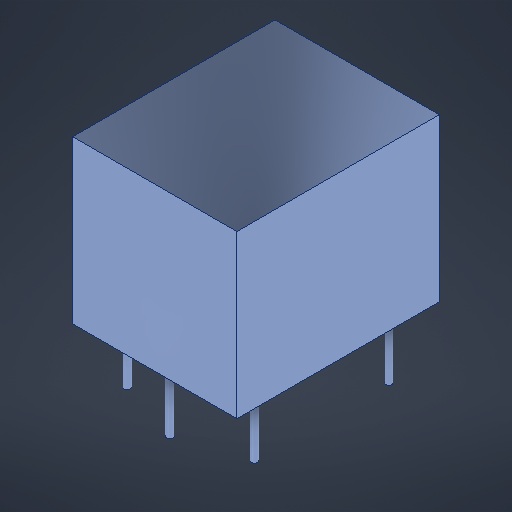
# Autodesk Inventor part: relay_sdr-03vdc-sl-c
Saved by Autodesk Inventor 2025.2 (Build 292293000, 293)
## iProperties
Created: 2025-11-15
Part Number: relay_sdr-03vdc-sl-c
Material: ABS Plastic
Document SubType Name: Modeling
Designer: sam
Density: 1.06 g/cm^3
Appearance: Cool Tint
Author: sam
Autodesk Inventor part; units mm, degrees
ref_plane "YZ Plane" through (0, 0, 0) normal (1, 0, 0) x (0, 1, 0)
ref_plane "XZ Plane" through (0, 0, 0) normal (0, 1, 0) x (-1, 0, 0)
ref_plane "XY Plane" through (0, 0, 0) normal (0, 0, 1) x (1, 0, 0)
sketch "Sketch1" plane through (0, 0, 0) normal (0, 1, 0) x (-1, 0, 0)
  line L0 (7.75, 9.55) -> (-7.75, 9.55)
  line L1 (-7.75, 9.55) -> (-7.75, -9.55)
  line L2 (-7.75, -9.55) -> (7.75, -9.55)
  line L3 (7.75, -9.55) -> (7.75, 9.55)
  line L4 (7.75, 9.55) -> (-7.75, -9.55) construction
  line L5 (-7.75, 9.55) -> (7.75, -9.55) construction
  point P0 (0, 0)
  dimension "d0" = 15.5
  dimension "d1" = 19.1
  constraints: 12 end point, 2 midpoint, 2 parallel, 1 horizontal, 1 perpendicular
  measures "d0" distance of L2.end L1.end
  measures "d1" distance of L1.end L0.end
extrude "Extrusion1" add sketch "Sketch1" along normal blind 15.3
sketch "Sketch2" plane through (0, 0, 0) normal (0, -1, 0) x (1, 0, 0)
  line L0 (7.75, 9.55) -> (7.75, -9.55) projected
  line L1 (-7.75, 9.55) -> (7.75, 9.55) projected
  line L2 (-7.75, -9.55) -> (-7.75, 9.55) projected
  line L3 (7.75, -9.55) -> (-7.75, -9.55) projected
  circle A0 centre (-6, 6.15) radius 0.3
  circle A1 centre (6, 6.15) radius 0.3
  circle A2 centre (0, 8.15) radius 0.3
  circle A3 centre (-6, -6.55) radius 0.3
  circle A4 centre (6, -6.55) radius 0.28
  point P0 (0, 0)
  dimension "d4" = 0.6
  dimension "d5" = 0.6
  dimension "d6" = 0.6
  dimension "d9" = 6
  dimension "d10" = 6
  dimension "d11" = 0.6
  dimension "d12" = 0.56
  dimension "d13" = 2
  dimension "d14" = 1.4
  dimension "d15" = 2
  dimension "d18" = 12.7
  dimension "d19" = 12.7
  constraints: 5 centre point
  measures "d4" diameter of A0
  measures "d5" diameter of A1
  measures "d6" diameter of A2
  measures "d9" horizontal distance of point (0, 0) A0.centre
  measures "d10" horizontal distance of A1.centre point (0, 0)
  measures "d11" diameter of A3
  measures "d12" diameter of A4
  measures "d13" vertical distance of A2.centre A0.centre
  measures "d14" distance from line of L1 A2.centre
  measures "d15" vertical distance of A2.centre A1.centre
  measures "d18" distance of A3.centre A0.centre
  measures "d19" distance of A4.centre A1.centre
extrude "Extrusion2" add sketch "Sketch2" along normal blind 6 contours A0 | A1 | A2 | A3 | A4
body "Solid1"
